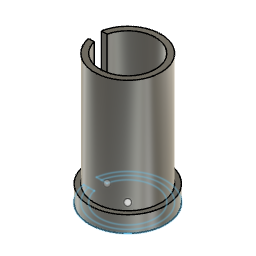
shim_half_inch_pipe (Autodesk Fusion 360 design; units mm, degrees)
Autodesk Fusion 360 part; units mm, degrees
sketch "Sketch1" plane through (0, 0, 0) normal (0, 0, 1) x (1, 0, 0)
  line L0 (-14.75, -2.5675) -> (-10.6089, -2.5675)
  line L1 (-10.6089, -2.5675) -> (-10.6082, -2.5702)
  line L2 (-10.6404, 2.5117) -> (-14.7873, 2.5117)
  arc A0 (-14.75, -2.5675) -> (-14.7873, 2.5117) centre (-0.0603, 0.0802) ccw
  arc A1 (-12.8266, -2.5675) -> (-12.8696, 2.5117) centre (-0.0603, 0.0802) ccw
  arc A2 (-10.6082, -2.5702) -> (-10.6589, 2.5117) centre (-0.0605, 0.0763) ccw
  constraint horizontal L0
  constraint horizontal L2
  constraint coincident L2 A1.end
  constraint coincident L0 A1.start
  constraint coincident L2 A2.end
sketch "Sketch3" plane through (0, 0, 0) normal (0, 0, 1) x (1, 0, 0)
extrude "Extrude1" add sketch "Sketch1" along normal blind 6.35
extrude "Extrude4" cut sketch "Sketch1" along normal blind 43.18 contours L0 L1 L2 A1 A2
extrude "Extrude5" add sketch "Sketch1" along normal blind 50.8 contours L0 L1 L2 A1 A2
extrude "Extrude3" [suppressed]
extrude "Extrude2" [suppressed]
